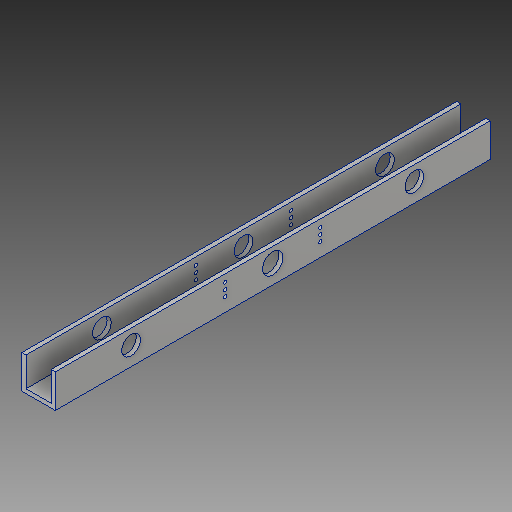
# Autodesk Inventor part: U
Saved by Autodesk Inventor 2018 (Build 220112000, 112)
## iProperties
Created: 2018-07-02
Part Number: U
Material: Aluminum 6061
Document SubType Name: Modeling
Designer: s-2512711
Density: 2.7 g/cm^3
Appearance: Aluminum - Flat
Author: s-2512711
Autodesk Inventor part; units mm, degrees
ref_plane "YZ Plane" through (0, 0, 0) normal (1, 0, 0) x (0, 1, 0)
ref_plane "XZ Plane" through (0, 0, 0) normal (0, 1, 0) x (-1, 0, 0)
ref_plane "XY Plane" through (0, 0, 0) normal (0, 0, 1) x (1, 0, 0)
sketch "Sketch1" plane through (0, 0, 0) normal (0, 0, 1) x (1, 0, 0)
  line L0 (0, 0) -> (6.35, 0)
  line L1 (6.35, 0) -> (6.35, 50.8)
  line L2 (6.35, 50.8) -> (0, 50.8)
  line L3 (0, 50.8) -> (0, 0)
  line L4 (0, 0) -> (50.8, 0)
  line L5 (50.8, 0) -> (50.8, 6.35)
  line L6 (50.8, 6.35) -> (0, 6.35)
  line L7 (0, 6.35) -> (0, 0)
  line L8 (50.8, 0) -> (44.45, 0)
  line L9 (44.45, 0) -> (44.45, 50.8)
  line L10 (44.45, 50.8) -> (50.8, 50.8)
  line L11 (50.8, 50.8) -> (50.8, 0)
  dimension "d0" = 6.35
  dimension "d1" = 50.8
  dimension "d2" = 50.8
  dimension "d3" = 6.35
  dimension "d4" = 6.35
  constraints: 24 end point, 6 parallel, 3 horizontal, 3 perpendicular
  measures "d0" distance of L2.end L1.end
  measures "d1" distance of L1.end L0.end
  measures "d2" distance of L6.end L5.end
  measures "d3" distance of L5.end L4.end
  measures "d4" distance of L9.end L10.end
extrude "Extrusion1" add sketch "Sketch1" along normal blind 660.4
sketch "Sketch2" plane through (50.8, 0, 0) normal (1, 0, 0) x (0, 0, -1)
  line L0 (0, 0) -> (0, 6.35)
  line L1 (0, 0) -> (0, 50.8) projected
  line L2 (0, 6.35) -> (-660.4, 6.35)
  line L3 (0, 0) -> (-660.4, 0) projected
  line L4 (0, 6.35) -> (0, 50.8) projected
  line L5 (0, 28.575) -> (-115.189, 28.575)
  circle A0 centre (-115.189, 28.575) radius 14.2875
  line L6 (-660.4, 6.35) -> (-660.4, 50.8) projected
  line L7 (-660.4, 28.575) -> (-545.211, 28.575)
  circle A1 centre (-545.211, 28.575) radius 14.2875
  line L8 (0, 50.8) -> (-660.4, 50.8) projected
  line L9 (-330.2, 50.8) -> (-330.2, 28.575)
  circle A2 centre (-330.2, 28.575) radius 14.2875
  dimension "d7" = 6.35
  dimension "d8" = 115.189
  dimension "d9" = 28.575
  dimension "d10" = 115.189
  dimension "d11" = 28.575
  constraints: 10 end point, 3 centre point, 3 coincident, 3 midpoint, 1 horizontal, 1 parallel, 1 perpendicular, 1 point on line, 1 vertical
  measures "d7" distance of L0.start L0.end
  measures "d8" distance of L5.start L5.end
  measures "d9" diameter of A0
  measures "d10" distance of L7.start L7.end
  measures "d11" diameter of A2
extrude "Extrusion2" cut sketch "Sketch2" against normal blind 660.4 contours A0 | A2 | A1
sketch "Sketch3" plane through (50.8, 0, 0) normal (1, 0, 0) x (0, 0, -1)
  circle A0 centre (-330.2, 28.575) radius 14.2875 projected
  circle A1 centre (-330.2, 28.575) radius 15.5575
  point P0 (0, 0)
  dimension "d14" = 31.115
  constraints: 1 centre point, 1 coincident
  measures "d14" diameter of A1
extrude "Extrusion3" cut sketch "Sketch3" against normal blind 25.4
sketch "Sketch4" plane through (50.8, 0, 0) normal (1, 0, 0) x (0, 0, -1)
  circle A0 centre (-330.2, 28.575) radius 15.5575 projected
  line L0 (-330.2, 28.575) -> (-330.2, 50.8)
  line L1 (0, 50.8) -> (-660.4, 50.8) projected
  line L2 (-330.2, 50.8) -> (-402.463, 50.8)
  line L3 (-402.463, 50.8) -> (-402.463, 39.6748)
  line L4 (-402.463, 39.6748) -> (-402.463, 30.1498)
  line L5 (-402.463, 30.1498) -> (-402.463, 20.6248)
  line L6 (-330.2, 50.8) -> (-257.937, 50.8)
  line L7 (-257.937, 50.8) -> (-257.937, 39.6748)
  line L8 (-257.937, 39.6748) -> (-257.937, 30.1498)
  line L9 (-257.937, 30.1498) -> (-257.937, 20.6248)
  circle A1 centre (-402.463, 39.6748) radius 2.54
  circle A2 centre (-402.463, 30.1498) radius 2.54
  circle A3 centre (-402.463, 20.6248) radius 2.54
  circle A4 centre (-257.937, 39.6748) radius 2.54
  circle A5 centre (-257.937, 30.1498) radius 2.54
  circle A6 centre (-257.937, 20.6248) radius 2.54
  point P0 (0, 0)
  dimension "d17" = 72.263
  dimension "d18" = 11.1252
  dimension "d19" = 9.525
  dimension "d20" = 9.525
  dimension "d21" = 72.263
  dimension "d22" = 5.08
  constraints: 18 end point, 6 centre point, 6 coincident, 6 point on line, 2 perpendicular, 1 midpoint
  measures "d17" distance of L0.end L2.end
  measures "d18" distance of L2.end L3.end
  measures "d19" distance of L3.end L4.end
  measures "d20" distance of L4.end L5.end
  measures "d21" distance of L0.end L6.end
  measures "d22" diameter of A1
extrude "Extrusion4" cut sketch "Sketch4" against normal blind 84.1375 contours A3 | A2 L5 L4 | L4 L5 A2 | A1 L4 L3 | L3 L4 A1 | A6 | A5 L9 L8 | L8 L9 A5 | A4 L8 L7 | L7 L8 A4
body "Solid1"
